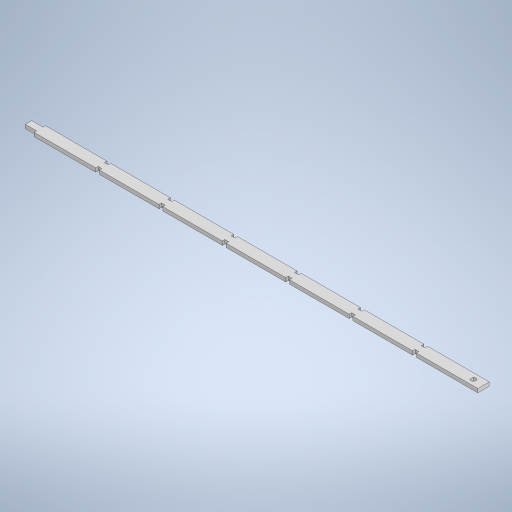
# Autodesk Inventor part: main_Bar
Saved by Autodesk Inventor 2024 (Build 280153000, 153)
## iProperties
Created: 2024-04-09
Part Number: main_Bar
Material: 一般
Document SubType Name: Modeling
Designer: USER
Density: 1 g/cm^3
Appearance: 預設
Author: USER
Autodesk Inventor part; units mm, degrees
ref_plane "YZ Plane" through (0, 0, 0) normal (1, 0, 0) x (0, 1, 0)
ref_plane "XZ Plane" through (0, 0, 0) normal (0, 1, 0) x (-1, 0, 0)
ref_plane "XY Plane" through (0, 0, 0) normal (0, 0, 1) x (1, 0, 0)
sketch "草圖1" plane through (0, 0, 0) normal (0, 1, 0) x (-1, 0, 0)
  line L0 (0, 0) -> (350, 0)
  line L1 (350, 0) -> (350, -9)
  line L2 (350, -9) -> (0, -9)
  line L3 (0, -9) -> (0, 0)
  arc A0 (9.5, -3.1771) -> (9.5, -5.8229) centre (8, -4.5) ccw
  line L4 (0, -4.5) -> (350, -4.5)
  line L5 (301.5, -9) -> (298.5, -9)
  line L6 (298.5, -9) -> (298.5, -7)
  line L7 (298.5, -7) -> (301.5, -7)
  line L8 (301.5, -7) -> (301.5, -9)
  line L9 (298.5, 0) -> (298.5, -2)
  line L10 (298.5, -2) -> (301.5, -2)
  line L11 (301.5, -2) -> (301.5, 0)
  line L12 (248.5, -9) -> (248.5, -7)
  line L13 (248.5, -7) -> (251.5, -7)
  line L14 (251.5, -7) -> (251.5, -9)
  line L15 (248.5, 0) -> (248.5, -2)
  line L16 (248.5, -2) -> (251.5, -2)
  line L17 (251.5, -2) -> (251.5, 0)
  line L18 (198.5, -9) -> (198.5, -7)
  line L19 (198.5, -7) -> (201.5, -7)
  line L20 (201.5, -7) -> (201.5, -9)
  line L21 (198.5, 0) -> (198.5, -2)
  line L22 (198.5, -2) -> (201.5, -2)
  line L23 (201.5, -2) -> (201.5, 0)
  line L24 (148.5, -9) -> (148.5, -7)
  line L25 (148.5, -7) -> (151.5, -7)
  line L26 (151.5, -7) -> (151.5, -9)
  line L27 (148.5, 0) -> (148.5, -2)
  line L28 (148.5, -2) -> (151.5, -2)
  line L29 (151.5, -2) -> (151.5, 0)
  line L30 (98.5, -9) -> (98.5, -7)
  line L31 (98.5, -7) -> (101.5, -7)
  line L32 (101.5, -7) -> (101.5, -9)
  line L33 (98.5, 0) -> (98.5, -2)
  line L34 (98.5, -2) -> (101.5, -2)
  line L35 (101.5, -2) -> (101.5, 0)
  line L36 (48.5, -9) -> (48.5, -7)
  line L37 (48.5, -7) -> (51.5, -7)
  line L38 (51.5, -7) -> (51.5, -9)
  line L39 (48.5, 0) -> (48.5, -2)
  line L40 (48.5, -2) -> (51.5, -2)
  line L41 (51.5, -2) -> (51.5, 0)
  line L42 (350, -2) -> (359, -2)
  line L43 (359, -2) -> (359, -7)
  line L44 (359, -7) -> (350, -7)
  line L45 (350, -7) -> (350, -2)
  line L46 (9.5, -3.1771) -> (9.5, -5.8229)
  point P0 (300, -9)
  point P1 (301.5, 0)
  point P2 (298.5, 0)
  point P3 (251.5, 0)
  point P4 (248.5, 0)
  point P5 (201.5, 0)
  point P6 (198.5, 0)
  point P7 (151.5, 0)
  point P8 (148.5, 0)
  point P9 (101.5, 0)
  point P10 (98.5, 0)
  point P11 (51.5, 0)
  point P12 (48.5, 0)
  point P13 (48.5, -9)
  point P14 (51.5, -9)
  point P15 (98.5, -9)
  point P16 (101.5, -9)
  point P17 (148.5, -9)
  point P18 (151.5, -9)
  point P19 (198.5, -9)
  point P20 (201.5, -9)
  point P21 (248.5, -9)
  point P22 (251.5, -9)
  point P23 (298.5, -9)
  point P24 (301.5, -9)
  dimension "d0" = 350
  dimension "d1" = 9
  dimension "d2" = 4
  dimension "d3" = 8
  dimension "d4" = 3
  dimension "d5" = 2
  dimension "d6" = 50
  dimension "d9" = 50
  dimension "d14" = 5
  dimension "d15" = 9
  dimension "d16" = 1.5
  constraints: 94 end point, 6 parallel, 4 horizontal, 4 midpoint, 4 symmetric about line, 3 perpendicular, 2 point on circle, 1 centre point, 1 horizontal alignment, 1 point on line, 1 vertical, 70 other
  measures "d0" distance of L1.end L2.end
  measures "d1" distance of L2.end L0.start
  measures "d2" diameter of A0
  measures "d3" distance from line of L3 A0.centre
  measures "d4" distance of L6.end L7.end
  measures "d5" distance of L7.end L5.start
  measures "d6" distance from line of L1 point (300, -9)
  measures "d9" distance of L6.end L12.end
  measures "d14" distance of L42.end L43.end
  measures "d15" distance of L43.end L44.end
  measures "d16" distance from line of A0.centre L46
extrude "擠出1" add sketch "草圖1" along normal blind 3 contours L0 L39 L40 L41 L33 L34 L35 L27 L28 L29 L21 L22 L23 L15 L16 L17 L9 L10 L11 L1 L4 L46 A0 L3 | L4 A0 L46 L1 L2 L8 L7 L6 L14 L13 L12 L20 L19 L18 L26 L25 L24 L32 L31 L30 L38 L37 L36 L3 | L1 L42 L43 L44
